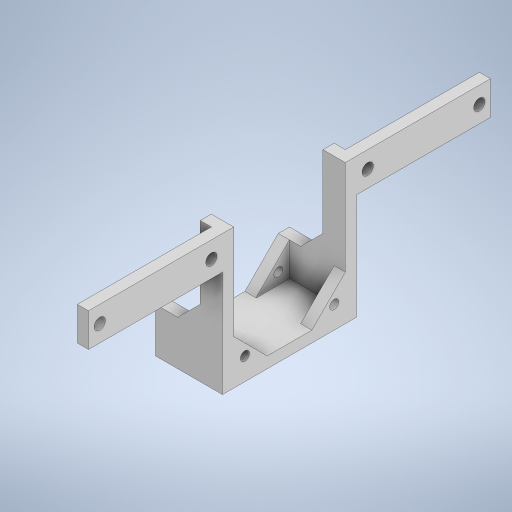
# Autodesk Inventor part: upper fan mount
Saved by Autodesk Inventor 2023 (Build 270158000, 158)
## iProperties
Created: 2023-05-15
Part Number: upper fan mount
Material: Generic
Document SubType Name: Modeling
Designer: skyfi
Density: 1 g/cm^3
Appearance: Default
Author: skyfi
Autodesk Inventor part; units mm, degrees
ref_plane "YZ Plane" through (0, 0, 0) normal (1, 0, 0) x (0, 1, 0)
ref_plane "XZ Plane" through (0, 0, 0) normal (0, 1, 0) x (-1, 0, 0)
ref_plane "XY Plane" through (0, 0, 0) normal (0, 0, 1) x (1, 0, 0)
sketch "Sketch1" plane through (0, 0, 0) normal (1, 0, 0) x (0, 1, 0)
  line L0 (15, 25) -> (-5, 25)
  line L1 (-5, 25) -> (-5, -25)
  line L2 (-5, -25) -> (15, -25)
  line L3 (15, -25) -> (0, -10)
  line L4 (0, -10) -> (0, 10)
  line L5 (0, 10) -> (15, 25)
  line L6 (0, 0) -> (-5, 0) construction
  circle A0 centre (5, -20) radius 2
  circle A1 centre (5, 20) radius 2
  dimension "d0" = 50
  dimension "d1" = 45
  dimension "d2" = 5
  dimension "d4" = 40
  dimension "d5" = 4
  dimension "d6" = 20
  dimension "d7" = 5
  dimension "d8" = 15
  constraints: 14 end point, 2 centre point, 2 equal length, 2 midpoint, 2 perpendicular, 1 coincident, 1 equal radius, 1 horizontal, 1 parallel, 1 vertical alignment
  measures "d0" distance of L0.end L1.end
  measures "d1" angle of L5 L0
  measures "d2" distance between parallel lines of L4 L1
  measures "d4" distance of A0.centre A1.centre
  measures "d5" diameter of A1
  measures "d6" vertical distance of point (0, 0) A0.centre
  measures "d7" distance from line of L4 A0.centre
  measures "d8" distance from line of L4 L2.end
extrude "Extrusion1" add sketch "Sketch1" along normal blind 5
sketch "Sketch2" plane through (0, 0, 0) normal (-1, 0, 0) x (0, 0, 1)
  line L0 (25, -5) -> (-25, -5) projected
  line L1 (-25, -5) -> (25, -5)
  line L2 (25, -5) -> (25, 0)
  line L3 (25, 0) -> (-25, 0)
  line L4 (-25, 0) -> (-25, -5)
  point P0 (0, 0)
  constraints: 8 end point, 2 parallel, 1 horizontal, 1 midpoint, 1 perpendicular
extrude "Extrusion2" add sketch "Sketch2" along normal blind 10
mirror "Mirror1" about plane through (-10, -2.5, 0) normal (-1, 0, 0)
sketch "Sketch5" plane through (5, -5, -25) normal (0, -1, 0) x (1, 0, 0)
  line L0 (0, 50) -> (0, 0) construction
  line L1 (0, 50) -> (-30, 50)
  line L2 (-30, 50) -> (-30, 55)
  line L3 (-30, 55) -> (0, 55)
  line L4 (0, 55) -> (0, 50)
  line L5 (-30, 0) -> (0, 0) projected
  line L6 (0, 0) -> (-30, 0)
  line L7 (-30, 0) -> (-30, -5)
  line L8 (-30, -5) -> (0, -5)
  line L9 (0, -5) -> (0, 0)
  line L10 (-30, 50) -> (-30, 0) construction
  point P0 (-5, 25)
  dimension "d19" = 5
  constraints: 16 end point, 4 parallel, 2 equal length, 2 horizontal, 2 perpendicular, 1 collinear
  measures "d19" distance of L3.end L0.start
extrude "Extrusion5" add sketch "Sketch5" against normal blind 62.5
sketch "Sketch6" plane through (-25, -5, 30) normal (0, 0, 1) x (1, 0, 0)
  line L0 (30, 62.5) -> (25, 62.5)
  line L1 (25, 62.5) -> (25, 47.5)
  line L2 (25, 47.5) -> (30, 47.5)
  line L3 (30, 47.5) -> (30, 62.5)
  line L4 (30, 0) -> (30, 62.5) construction
  dimension "d25" = 5
  dimension "d26" = 15
  constraints: 9 end point, 2 parallel, 1 horizontal, 1 perpendicular
  measures "d25" distance of L0.start L0.end
  measures "d26" distance of L0.end L1.end
extrude "Extrusion6" add sketch "Sketch6" along normal blind 60
sketch "Sketch8" plane through (5, 0, 0) normal (1, 0, 0) x (0, 0, -1)
  line L0 (-30, 42.5) -> (-30, 57.5) construction
  line L1 (-30, 50) -> (-90, 50) construction
  line L2 (-90, 42.5) -> (-90, 57.5) construction
  circle A0 centre (-85, 50) radius 2.5
  circle A1 centre (-35, 50) radius 2.5
  point P0 (0, 0)
  dimension "d31" = 5
  dimension "d32" = 5
  dimension "d33" = 5
  constraints: 2 centre point, 2 end point, 2 midpoint, 2 point on line, 1 equal radius
  measures "d31" diameter of A0
  measures "d32" distance from line of A0.centre L2
  measures "d33" distance from line of L0 A1.centre
extrude "Extrusion8" cut sketch "Sketch8" against normal blind 10
mirror "Mirror2" about plane through (0, 0, 0) normal (0, 0, 1) of "Extrusion6", "Extrusion8"
sketch "Sketch7" plane through (-25, -5, 30) normal (0, 0, 1) x (1, 0, 0)
  line L0 (0, 62.5) -> (25, 62.5) construction
  line L1 (0, 0) -> (0, 62.5) construction
  line L2 (0, 62.5) -> (0, 20)
  line L3 (0, 20) -> (0, 62.5) projected
  line L4 (0, 20) -> (10, 20)
  line L5 (10, 20) -> (20, 30)
  line L6 (0, 20) -> (0, 62.5) projected
  line L7 (0, 62.5) -> (20, 62.5)
  line L8 (20, 30) -> (20, 62.5)
  line L9 (30, 62.5) -> (0, 62.5) construction
  line L10 (25, 47.5) -> (25, 62.5) projected
  point P0 (25, 5)
  dimension "d38" = 5
  dimension "d39" = 45
  dimension "d40" = 10
  constraints: 10 end point, 1 horizontal, 1 perpendicular, 1 point on line
  measures "d38" distance between parallel lines of L10 L8
  measures "d39" angle of L2 L5
  measures "d40" distance of L2.end L4.end
extrude "Extrusion7" cut sketch "Sketch7" along normal through all both and the other way through all
sketch "Sketch3" plane through (0, 0, 10) normal (0, 1, 0) x (1, 0, 0)
  line L0 (-20, 0) -> (-20, -15) construction
  line L1 (0, 20) -> (5, 20) construction
  line L2 (-20, 0) -> (0, 20) construction
  line L3 (-20, 35) -> (-20, 20) construction
  line L4 (0, 0) -> (5, 0) construction
  line L5 (-20, 20) -> (0, 0) construction
  circle A0 centre (-10, 10) radius 3
  point P0 (0, 10)
  dimension "d13" = 6
  constraints: 4 end point, 1 centre point, 1 midpoint
  measures "d13" diameter of A0
sketch "Sketch4" plane through (0, 0, 10) normal (0, 1, 0) x (1, 0, 0)
  circle A0 centre (-10, 10) radius 3 projected
  circle A1 centre (-10, 10) radius 2
  point P0 (0, 10)
  dimension "d16" = 4
  constraints: 1 centre point, 1 coincident
  measures "d16" diameter of A1
equation "\"d6\" = 0.5 * d4"
equation "\"d7\" = 0.333333 * d8"
body "Solid1"
